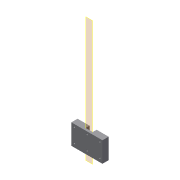
# Autodesk Inventor part: 04_Mount_Rail_Fastener
Saved by Autodesk Inventor 2019.4 (Build 234330000, 330)
## iProperties
Created: 2021-02-16
Part Number: 04_Mount_Rail_Fastener
Material: Generic
Document SubType Name: Modeling
Designer: diederichbenedict
Density: 1 g/cm^3
Appearance: Default
Author: diederichbenedict
Autodesk Inventor part; units mm, degrees
ref_plane "YZ Plane" through (0, 0, 0) normal (1, 0, 0) x (0, 1, 0)
ref_plane "XZ Plane" through (0, 0, 0) normal (0, 1, 0) x (-1, 0, 0)
ref_plane "XY Plane" through (0, 0, 0) normal (0, 0, 1) x (1, 0, 0)
ref_plane "Work Plane1" through (22.0339, 196.5, 8) normal (0, 0, 1) x (1, 0, 0)
sketch "Sketch1" plane through (22.0339, 196.5, 8) normal (0, 0, 1) x (1, 0, 0)
  circle A0 centre (5.4838, -190) radius 1.4 projected
  circle A1 centre (27.9838, -190) radius 1.4 projected
  circle A2 centre (-17.0162, -190) radius 1.4 projected
  line L0 (-22.0339, -196.5) -> (32.9661, -196.5) projected
  line L1 (32.9661, -196.5) -> (32.9661, -186.5) projected
  line L2 (-22.0339, -186.5) -> (32.9661, -186.5) projected
  line L3 (-22.0339, -196.5) -> (-22.0339, -186.5) projected
  circle A3 centre (27.9838, -165) radius 1.4 projected
  circle A4 centre (-17.0162, -165) radius 1.4 projected
  circle A5 centre (5.4838, -165) radius 1.4 projected
  line L4 (32.9661, -160.5) -> (32.9661, -169.5) projected
  line L5 (-22.0339, -160.5) -> (32.9661, -160.5) projected
  line L6 (-22.0339, -160.5) -> (-22.0339, -169.5) projected
  line L7 (32.9661, -169.5) -> (-22.0339, -169.5) projected
  line L8 (32.9661, -196.5) -> (-22.0339, -196.5)
  line L9 (-22.0339, -196.5) -> (-22.0339, -160.5)
  line L10 (-22.0339, -160.5) -> (32.9661, -160.5)
  line L11 (32.9661, -160.5) -> (32.9661, -196.5)
  constraints: 8 end point, 2 parallel, 1 horizontal, 1 perpendicular
extrude "Extrusion1" add sketch "Sketch1" along normal blind 4
sketch "Sketch2" plane through (22.0339, 196.5, 8) normal (0, 0, -1) x (-1, 0, 0)
  circle A0 centre (17.0162, -190) radius 1.4 projected
  circle A1 centre (-27.9838, -190) radius 1.4 projected
  circle A2 centre (-5.4838, -190) radius 1.4 projected
  circle A3 centre (-5.4838, -165) radius 1.4 projected
  circle A4 centre (17.0162, -165) radius 1.4 projected
  circle A5 centre (-27.9838, -165) radius 1.4 projected
  line L0 (-32.9661, -196.5) -> (-32.9661, -160.5) projected
  line L1 (22.0339, -196.5) -> (-32.9661, -196.5) projected
  line L2 (22.0339, -160.5) -> (22.0339, -196.5) projected
  line L3 (-32.9661, -160.5) -> (22.0339, -160.5) projected
  line L4 (22.0339, -196.5) -> (-32.9661, -196.5) projected
  line L5 (22.0339, -160.5) -> (0.6985, -160.5)
  line L6 (0.6985, -160.5) -> (0.6985, -196.5)
  line L7 (0.6985, -196.5) -> (22.0339, -196.5)
  line L8 (22.0339, -196.5) -> (22.0339, -160.5)
  line L9 (-32.9661, -196.5) -> (-32.9661, -160.5) projected
  line L10 (-32.9661, -160.5) -> (-11.6661, -160.5)
  line L11 (-11.6661, -160.5) -> (-11.6661, -196.5)
  line L12 (-11.6661, -196.5) -> (-32.9661, -196.5)
  line L13 (-32.9661, -196.5) -> (-32.9661, -160.5)
  line L14 (-11.4661, 0) -> (-11.4661, -200) projected
  line L15 (0.4985, 0) -> (0.4985, -200) projected
  dimension "d6" = 0.2
  dimension "d7" = 0.2
  constraints: 16 end point, 4 parallel, 2 horizontal, 2 perpendicular, 2 point on line
  measures "d6" distance between parallel lines of L15 L6
  measures "d7" distance between parallel lines of L14 L11
extrude "Extrusion2" add sketch "Sketch2" along normal blind 7 contours L0 L3 L11 L1 | L6 L3 L2 L1
body "Solid1"
